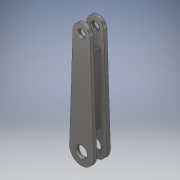
# Autodesk Inventor part: Lower Rocker Arm Spider Crab
Saved by Autodesk Inventor 2019 (Build 230136000, 136)
## iProperties
Created: 2019-08-25
Part Number: Lower Rocker Arm Spider Crab
Material: Steel, Mild
Document SubType Name: Modeling
Designer: DIBYOJYOTI
Density: 7.85 g/cm^3
Appearance: Semi-Polished
Mass: 56.6792 g
Surface Area: 34.608 cm^2
Volume: 7.92716 cm^3
Author: DIBYOJYOTI
Autodesk Inventor part; units mm, degrees
ref_plane "YZ Plane" through (0, 0, 0) normal (1, 0, 0) x (0, 1, 0)
ref_plane "XZ Plane" through (0, 0, 0) normal (0, 1, 0) x (-1, 0, 0)
ref_plane "XY Plane" through (0, 0, 0) normal (0, 0, 1) x (1, 0, 0)
sketch "Sketch1" plane through (0, 0, 0) normal (0, 0, 1) x (1, 0, 0)
  circle A0 centre (0, 0) radius 3.05
  arc A1 (-6.9961, 0.2328) -> (6.9961, 0.2339) centre (0, 0) ccw
  circle A2 centre (-0.0048, 60) radius 2.05
  arc A3 (4.9924, 60.1671) -> (-5.002, 60.1663) centre (-0.0048, 60) ccw
  line L0 (-5.002, 60.1663) -> (-6.9961, 0.2328)
  line L1 (4.9924, 60.1671) -> (6.9961, 0.2339)
  line L2 (-3, 10) -> (3, 10)
  line L3 (3, 10) -> (3, 50)
  line L4 (3, 50) -> (-3, 50)
  line L5 (-3, 50) -> (-3, 10)
  point P0 (-7, 0)
  dimension "d0" = 6.1
  dimension "d1" = 14
  dimension "d3" = 4.1
  dimension "d4" = 10
  dimension "d5" = 60
  dimension "d18" = 6
  dimension "d19" = 40
  constraints: 12 end point, 5 point on circle, 4 centre point, 4 tangent, 3 coincident, 2 parallel, 1 horizontal, 1 perpendicular
  measures "d0" diameter of A0
  measures "d1" diameter of A1
  measures "d3" diameter of A2
  measures "d4" diameter of A3
  measures "d5" distance of point (0, 0) A2.centre
  measures "d18" distance of L4.end L3.end
  measures "d19" distance of L3.end L2.end
extrude "Extrusion1" add sketch "Sketch1" along normal blind 8 and the other way blind 2 contours L0 A3 L1 A1 | L5 L4 L3 L2
fillet "Fillet1" radius 0.5 4 edges at (-3.05, 0, 8) (-3.05, 0, -2) (-2.0548, 60, -2) (-2.0548, 60, 8) curvature continuous yes
shell "Shell1" thickness 2 removed faces 4 at (-5.6667, 40.1884, 4.6667) at (5.6603, 40.1893, 1.3333) at (-6.9398, -0.9162, 4.6667) at (-2.4569, 64.3574, 4.6667)
extrude "Extrusion2" add sketch "Sketch1" along normal blind 6 contours L5 L4 L3 L2
delete faces "Delete Face1" heal yes whole lump no faces at (4.0321, 60.3259, 2) (2.0187, 59.6712, 4.5) (5.0336, 0.4064, 2) (3.0105, -0.4893, 4.5)
fillet "Fillet2" radius 0.5 4 edges at (-2.0548, 60, 6) (-2.0548, 60, 0) (-3.05, 0, 0) (-3.05, 0, 6) curvature continuous yes
body "Solid1"
